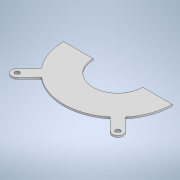
# Autodesk Inventor part: Rail
Saved by Autodesk Inventor 2022.2 (Build 262287010, 287A)
## iProperties
Created: 2022-03-31
Part Number: Rail
Material: Genérico
Document SubType Name: Modeling
Designer: mabel
Density: 1 g/cm^3
Appearance: Valor por defecto
Author: mabel
Autodesk Inventor part; units mm, degrees
ref_plane "YZ Plane" through (0, 0, 0) normal (1, 0, 0) x (0, 1, 0)
ref_plane "XZ Plane" through (0, 0, 0) normal (0, 1, 0) x (-1, 0, 0)
ref_plane "XY Plane" through (0, 0, 0) normal (0, 0, 1) x (1, 0, 0)
sketch "Boceto1" plane through (0, 0, 0) normal (0, 1, 0) x (-1, 0, 0)
  arc A0 (30.25, 0) -> (-30.25, 0) centre (0, 0) ccw
  circle A1 centre (0, 0) radius 81.4 construction
  line L0 (66, 0) -> (30.25, 0)
  line L1 (-30.25, 0) -> (-66, 0)
  line L2 (0, 0) -> (103.5194, 0) construction
  line L3 (73.1993, 73.1993) -> (0, 0) construction
  line L4 (0, 0) -> (-73.1993, 73.1993) construction
  line L5 (0, 0) -> (103.5194, 0) construction
  line L6 (66, 66) -> (36.5996, 36.5996) construction
  line L7 (56.6662, 66) -> (41.7682, 51.102)
  line L8 (51.102, 41.7682) -> (66, 56.6662)
  arc A2 (66, 56.6662) -> (56.6662, 66) centre (61.3331, 61.3331) ccw
  line L9 (0, 0) -> (0, 91.3472) construction
  line L10 (-56.6662, 66) -> (-41.7682, 51.102)
  line L11 (-51.102, 41.7682) -> (-66, 56.6662)
  arc A3 (-56.6662, 66) -> (-66, 56.6662) centre (-61.3331, 61.3331) ccw
  circle A4 centre (61.3331, 61.3331) radius 2.75
  circle A5 centre (-61.3331, 61.3331) radius 2.75
  arc A6 (66, 0) -> (51.102, 41.7682) centre (0, 0) ccw
  arc A7 (41.7682, 51.102) -> (-41.7682, 51.102) centre (0, 0) ccw
  arc A8 (-51.102, 41.7682) -> (-66, 0) centre (0, 0) ccw
  point P0 (36.5996, 45.9334)
  point P1 (45.9334, 36.5996)
  point P2 (51.2998, 51.2998)
  point P3 (-36.5996, 45.9334)
  point P4 (-45.9334, 36.5996)
  dimension "d9" = 5.5
  dimension "d11" = 5.5
  constraints: 26 end point, 13 point on circle, 9 centre point, 5 symmetric about line, 4 coincident, 4 horizontal, 2 midpoint, 2 point on line, 2 tangent, 1 equal length, 1 parallel, 1 vertical, 1 other
  measures "d9" diameter of A4
  measures "d11" diameter of A5
extrude "Extrusión2" add sketch "Boceto1" along normal blind 2
